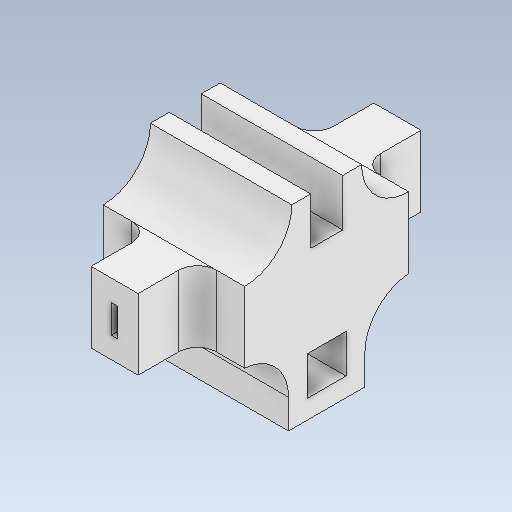
# Autodesk Inventor part: fuselage_wing_interface_v2
Saved by Autodesk Inventor 2021 (Build 250183000, 183)
## iProperties
Created: 2020-11-15
Part Number: fuselage_wing_interface_v2
Material: ABS Plastic
Document SubType Name: Modeling
Designer: Paco
Density: 1.06 g/cm^3
Appearance: Smooth - White
Mass: 3.97143 g
Surface Area: 23.6284 cm^2
Volume: 3.74663 cm^3
Author: Paco
Autodesk Inventor part; units mm, degrees
ref_plane "YZ Plane" through (0, 0, 0) normal (1, 0, 0) x (0, 1, 0)
ref_plane "XZ Plane" through (0, 0, 0) normal (0, 1, 0) x (-1, 0, 0)
ref_plane "XY Plane" through (0, 0, 0) normal (0, 0, 1) x (1, 0, 0)
sketch "Sketch1" plane through (0, 0, 0) normal (1, 0, 0) x (0, 1, 0)
  line L0 (4.05, 4.05) -> (-4.05, 4.05)
  line L1 (-4.05, 4.05) -> (-4.05, -4.05)
  line L2 (-4.05, -4.05) -> (4.05, -4.05)
  line L3 (4.05, -4.05) -> (4.05, 4.05)
  line L4 (11.55, 15) -> (4.05, 15)
  line L5 (4.05, 15) -> (4.05, -15)
  line L6 (4.05, -15) -> (11.55, -15)
  line L7 (11.55, -15) -> (11.55, 15)
  line L8 (4.05, 4.05) -> (-4.05, -4.05) construction
  line L9 (4.05, -4.05) -> (-4.05, 4.05) construction
  line L10 (2.05, 2.05) -> (-2.05, 2.05)
  line L11 (-2.05, 2.05) -> (-2.05, -2.05)
  line L12 (-2.05, -2.05) -> (2.05, -2.05)
  line L13 (2.05, -2.05) -> (2.05, 2.05)
  line L14 (2.05, 2.05) -> (-2.05, -2.05) construction
  line L15 (-2.05, 2.05) -> (2.05, -2.05) construction
  point P0 (4.05, 4.05)
  point P1 (0, 0)
  point P2 (0, 0)
  point P3 (0, 0)
  dimension "d0" = 8.1
  dimension "d3" = 8.1
  dimension "d22" = 10.95
  dimension "d24" = 30
  dimension "d25" = 7.5
  dimension "d55" = 10.95
  dimension "d65" = 4.1
  dimension "d66" = 4.1
  constraints: 32 end point, 6 parallel, 4 midpoint, 4 perpendicular, 3 horizontal, 1 coincident, 1 collinear, 1 point on line, 1 other
  measures "d0" distance of L2.end L0.start
  measures "d3" distance of L1.end L2.end
  measures "d22" distance between parallel lines of L0 L4
  measures "d24" distance of L6.end L4.start
  measures "d25" distance of L5.end L6.end
  measures "d55" distance between parallel lines of L2 L6
  measures "d65" distance of L12.end L10.start
  measures "d66" distance of L11.end L12.end
extrude "Extrusion1" add sketch "Sketch1" along normal blind 15
sketch "Sketch5" plane through (0, 4.05, 15) normal (0, 0, 1) x (1, 0, 0)
  line L0 (7.15, 5.25) -> (7.85, 5.25)
  line L1 (7.85, 5.25) -> (7.85, 2.25)
  line L2 (7.85, 2.25) -> (7.15, 2.25)
  line L3 (7.15, 2.25) -> (7.15, 5.25)
  line L4 (0, 0) -> (15, 0) projected
  line L5 (0, 7.5) -> (0, 0) projected
  point P0 (0, -4.05)
  dimension "d86" = 3
  dimension "d87" = 0.7
  dimension "d88" = 2.25
  dimension "d89" = 7.15
  constraints: 8 end point, 2 parallel, 1 horizontal, 1 perpendicular
  measures "d86" distance of L0.end L1.end
  measures "d87" distance of L1.end L2.end
  measures "d88" distance between parallel lines of L4 L2
  measures "d89" distance between parallel lines of L5 L3
extrude "Extrusion4" cut sketch "Sketch5" against normal through all
fillet "Fillet3" radius 5 2 edges at (7.5, 4.05, 4.05) (7.5, 4.05, -4.05)
sketch "Sketch7" plane through (0, 0, 0) normal (-1, 0, 0) x (0, 0, 1)
  line L0 (3.7, 11.55) -> (1.7, 11.55)
  line L1 (1.7, 11.55) -> (1.7, 16.55)
  line L2 (1.7, 16.55) -> (3.7, 16.55)
  line L3 (3.7, 16.55) -> (3.7, 11.55)
  line L4 (3.7, 11.55) -> (1.7, 16.55) construction
  line L5 (1.7, 11.55) -> (3.7, 16.55) construction
  line L6 (-1.7, 11.55) -> (-3.7, 11.55)
  line L7 (-3.7, 11.55) -> (-3.7, 16.55)
  line L8 (-3.7, 16.55) -> (-1.7, 16.55)
  line L9 (-1.7, 16.55) -> (-1.7, 11.55)
  line L10 (-1.7, 11.55) -> (-3.7, 16.55) construction
  line L11 (-3.7, 11.55) -> (-1.7, 16.55) construction
  line L12 (-15, 11.55) -> (15, 11.55) projected
  point P0 (0, 0)
  point P1 (2.7, 14.05)
  point P2 (-2.7, 14.05)
  dimension "d77" = 5
  dimension "d78" = 2
  dimension "d79" = 2
  dimension "d80" = 3.4
  dimension "d82" = 1.7
  constraints: 24 end point, 4 midpoint, 4 parallel, 3 collinear, 2 horizontal, 2 perpendicular
  measures "d77" distance of L2.end L0.start
  measures "d78" distance of L7.end L8.end
  measures "d79" distance of L1.end L2.end
  measures "d80" distance between parallel lines of L9 L1
  measures "d82" distance from line of L1 point (0, 0)
extrude "Extrusion5" add sketch "Sketch7" against normal up to surface (15 mm away)
fillet "Fillet4" radius 5 2 edges at (7.5, 11.55, 3.7) (7.5, 11.55, -3.7)
sketch "Sketch8" plane through (0, 11.55, -15) normal (0, 1, 0) x (1, 0, 0)
  line L0 (0, -23.7) -> (15, -23.7) projected
  line L1 (15, -30) -> (10, -30)
  line L2 (10, -30) -> (10, -23.7)
  line L3 (10, -23.7) -> (15, -23.7)
  line L4 (15, -23.7) -> (15, -30)
  line L5 (0, -30) -> (5, -30)
  line L6 (5, -30) -> (5, -23.7)
  line L7 (5, -23.7) -> (0, -23.7)
  line L8 (0, -23.7) -> (0, -30)
  line L9 (0, -5.95) -> (0, 0) projected
  line L10 (0, 0) -> (5, 0)
  line L11 (5, 0) -> (5, -6.3)
  line L12 (5, -6.3) -> (0, -6.3)
  line L13 (0, -6.3) -> (0, 0)
  line L14 (15, -6.3) -> (0, -6.3) projected
  line L15 (15, -5.95) -> (15, 0) projected
  line L16 (10, -6.3) -> (15, -6.3)
  line L17 (15, -6.3) -> (15, 0)
  line L18 (15, 0) -> (10, 0)
  line L19 (10, 0) -> (10, -6.3)
  point P0 (0, -15)
  dimension "d90" = 5
  dimension "d91" = 5
  dimension "d92" = 5
  dimension "d93" = 5
  constraints: 32 end point, 8 parallel, 4 horizontal, 4 perpendicular, 3 point on line
  measures "d90" distance of L5.start L5.end
  measures "d91" distance of L1.start L1.end
  measures "d92" distance of L11.end L12.end
  measures "d93" distance of L16.start L16.end
extrude "Extrusion6" cut sketch "Sketch8" against normal blind 10
fillet "Fillet5" radius 2 4 edges at (5, 7.7939, 8.7) (10, 7.7939, 8.7) (10, 7.7939, -8.7) (5, 7.7939, -8.7)
equation "\"d3\" = d0"
equation "\"d22\" = d55"
body "Solid1"
